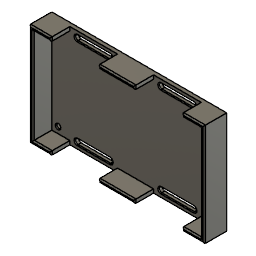
chassis_layer1_assembly_check_v0_1 (Autodesk Fusion 360 archive; units mm, degrees)
design "power_tray_v0_1_fusion_final"
part number: 2026-05-26-08-43-21-523
Autodesk Fusion 360 part; units mm, degrees
sketch "草图12" plane through (0, 0, 0) normal (0, 0, 1) x (1, 0, 0)
  line L0 (-69.75, -40.85) -> (69.75, -40.85)
  line L1 (69.75, -40.85) -> (69.75, 40.85)
  line L2 (69.75, 40.85) -> (-69.75, 40.85)
  line L3 (-69.75, 40.85) -> (-69.75, -40.85)
extrude "拉伸12" add sketch "草图12" along normal blind 3
ref_plane "工作平面2" through (0, 0, 3) normal (0, 0, 1) x (1, 0, 0)
sketch "草图13" plane through (0, 0, 3) normal (0, 0, 1) x (1, 0, 0)
  line L0 (-69.75, -40.85) -> (-66.75, -40.85)
  line L1 (-66.75, -40.85) -> (-66.75, 40.85)
  line L2 (-66.75, 40.85) -> (-69.75, 40.85)
  line L3 (-69.75, 40.85) -> (-69.75, -40.85)
extrude "拉伸13" add sketch "草图13" along normal blind 15
sketch "草图14" plane through (0, 0, 3) normal (0, 0, 1) x (1, 0, 0)
  line L0 (66.75, -40.85) -> (69.75, -40.85)
  line L1 (69.75, -40.85) -> (69.75, 40.85)
  line L2 (69.75, 40.85) -> (66.75, 40.85)
  line L3 (66.75, 40.85) -> (66.75, -40.85)
extrude "拉伸14" add sketch "草图14" along normal blind 15
sketch "草图15" plane through (0, 0, 3) normal (0, 0, 1) x (1, 0, 0)
  line L0 (-66.75, -40.85) -> (-52.375, -40.85)
  line L1 (-52.375, -40.85) -> (-52.375, -37.85)
  line L2 (-52.375, -37.85) -> (-66.75, -37.85)
  line L3 (-66.75, -37.85) -> (-66.75, -40.85)
extrude "拉伸15" add sketch "草图15" along normal blind 15
sketch "草图16" plane through (0, 0, 3) normal (0, 0, 1) x (1, 0, 0)
  line L0 (-14.375, -40.85) -> (14.375, -40.85)
  line L1 (14.375, -40.85) -> (14.375, -37.85)
  line L2 (14.375, -37.85) -> (-14.375, -37.85)
  line L3 (-14.375, -37.85) -> (-14.375, -40.85)
extrude "拉伸16" add sketch "草图16" along normal blind 15
sketch "草图17" plane through (0, 0, 3) normal (0, 0, 1) x (1, 0, 0)
  line L0 (52.375, -40.85) -> (66.75, -40.85)
  line L1 (66.75, -40.85) -> (66.75, -37.85)
  line L2 (66.75, -37.85) -> (52.375, -37.85)
  line L3 (52.375, -37.85) -> (52.375, -40.85)
extrude "拉伸17" add sketch "草图17" along normal blind 15
sketch "草图18" plane through (0, 0, 3) normal (0, 0, 1) x (1, 0, 0)
  line L0 (-66.75, 37.85) -> (-52.375, 37.85)
  line L1 (-52.375, 37.85) -> (-52.375, 40.85)
  line L2 (-52.375, 40.85) -> (-66.75, 40.85)
  line L3 (-66.75, 40.85) -> (-66.75, 37.85)
extrude "拉伸18" add sketch "草图18" along normal blind 15
sketch "草图19" plane through (0, 0, 3) normal (0, 0, 1) x (1, 0, 0)
  line L0 (-14.375, 37.85) -> (14.375, 37.85)
  line L1 (14.375, 37.85) -> (14.375, 40.85)
  line L2 (14.375, 40.85) -> (-14.375, 40.85)
  line L3 (-14.375, 40.85) -> (-14.375, 37.85)
extrude "拉伸19" add sketch "草图19" along normal blind 15
sketch "草图20" plane through (0, 0, 3) normal (0, 0, 1) x (1, 0, 0)
  line L0 (52.375, 37.85) -> (66.75, 37.85)
  line L1 (66.75, 37.85) -> (66.75, 40.85)
  line L2 (66.75, 40.85) -> (52.375, 40.85)
  line L3 (52.375, 40.85) -> (52.375, 37.85)
extrude "拉伸20" add sketch "草图20" along normal blind 15
sketch "草图21" plane through (0, 0, 3) normal (0, 0, 1) x (1, 0, 0)
  line L0 (-46.375, -33.85) -> (-20.375, -33.85)
  line L1 (-20.375, -37.85) -> (-46.375, -37.85)
  arc A0 (-20.375, -37.85) -> (-20.375, -33.85) centre (-20.375, -35.85) ccw
  arc A1 (-46.375, -33.85) -> (-46.375, -37.85) centre (-46.375, -35.85) ccw
  line L2 (-46.375, 37.85) -> (-20.375, 37.85)
  line L3 (-20.375, 33.85) -> (-46.375, 33.85)
  arc A2 (-20.375, 33.85) -> (-20.375, 37.85) centre (-20.375, 35.85) ccw
  arc A3 (-46.375, 37.85) -> (-46.375, 33.85) centre (-46.375, 35.85) ccw
  line L4 (20.375, -33.85) -> (46.375, -33.85)
  line L5 (46.375, -37.85) -> (20.375, -37.85)
  arc A4 (46.375, -37.85) -> (46.375, -33.85) centre (46.375, -35.85) ccw
  arc A5 (20.375, -33.85) -> (20.375, -37.85) centre (20.375, -35.85) ccw
  line L6 (20.375, 37.85) -> (46.375, 37.85)
  line L7 (46.375, 33.85) -> (20.375, 33.85)
  arc A6 (46.375, 33.85) -> (46.375, 37.85) centre (46.375, 35.85) ccw
  arc A7 (20.375, 37.85) -> (20.375, 33.85) centre (20.375, 35.85) ccw
extrude "拉伸21" cut sketch "草图21" against normal blind 3.2
sketch "草图22" plane through (0, 0, 3) normal (0, 0, 1) x (1, 0, 0)
  circle A0 centre (-61.75, -32.85) radius 1.6
  circle A1 centre (-61.75, 32.85) radius 1.6
  circle A2 centre (61.75, -32.85) radius 1.6
  circle A3 centre (61.75, 32.85) radius 1.6
extrude "拉伸22" cut sketch "草图22" against normal blind 3.2
fillet "圆角2" radius 1 24 edges at (59.5625, 37.85, 18) (52.375, 39.35, 18) (66.75, 0, 18) (14.375, 39.35, 18) (0, 37.85, 18) (-14.375, 39.35, 18) (0, 40.85, 18) (-52.375, 39.35, 18) (-59.5625, 37.85, 18) (59.5625, -37.85, 18) (52.375, -39.35, 18) (0, -37.85, 18) (14.375, -39.35, 18) (-14.375, -39.35, 18) (0, -40.85, 18) (-59.5625, -37.85, 18) (-52.375, -39.35, 18) (-66.75, 0, 18) (61.0625, -40.85, 18) (69.75, 0, 18) (61.0625, 40.85, 18) (-69.75, 0, 18) (-61.0625, -40.85, 18) (-61.0625, 40.85, 18)
fillet "圆角3" radius 0.6 68 edges at (60.2583, -32.2714, 3) (-63.2417, 33.4286, 3) (-63.2417, -32.2714, 3) (60.2583, 33.4286, 3) (33.375, -37.85, 3) (18.375, -35.85, 3) (33.375, -33.85, 3) (48.375, -35.85, 3) (48.375, -35.85, 3) (33.375, -37.85, 3) (18.375, -35.85, 3) (33.375, -33.85, 3) (33.375, -33.85, 3) (48.375, -35.85, 3) (33.375, -37.85, 3) (18.375, -35.85, 3) (18.375, -35.85, 3) (33.375, -33.85, 3) (48.375, -35.85, 3) (33.375, -37.85, 3) (-33.375, 33.85, 3) (-48.375, 35.85, 3) (-33.375, 37.85, 3) (-18.375, 35.85, 3) (-18.375, 35.85, 3) (-33.375, 33.85, 3) (-48.375, 35.85, 3) (-33.375, 37.85, 3) (-33.375, 37.85, 3) (-18.375, 35.85, 3) (-33.375, 33.85, 3) (-48.375, 35.85, 3) (-48.375, 35.85, 3) (-33.375, 37.85, 3) (-18.375, 35.85, 3) (-33.375, 33.85, 3) (-33.375, -37.85, 3) (-48.375, -35.85, 3) (-33.375, -33.85, 3) (-18.375, -35.85, 3) (-18.375, -35.85, 3) (-33.375, -37.85, 3) (-48.375, -35.85, 3) (-33.375, -33.85, 3) (-33.375, -33.85, 3) (-18.375, -35.85, 3) (-33.375, -37.85, 3) (-48.375, -35.85, 3) (-48.375, -35.85, 3) (-33.375, -33.85, 3) (-18.375, -35.85, 3) (-33.375, -37.85, 3) (33.375, 33.85, 3) (18.375, 35.85, 3) (33.375, 37.85, 3) (48.375, 35.85, 3) (48.375, 35.85, 3) (33.375, 33.85, 3) (18.375, 35.85, 3) (33.375, 37.85, 3) (33.375, 37.85, 3) (48.375, 35.85, 3) (33.375, 33.85, 3) (18.375, 35.85, 3) (18.375, 35.85, 3) (33.375, 37.85, 3) (48.375, 35.85, 3) (33.375, 33.85, 3)
sketch "草图7" plane through (0, 0, 3) normal (0, 0, 1) x (1, 0, 0)
  line L0 (-66.75, 37.85) -> (-52.375, 37.85)
  line L1 (-52.375, 37.85) -> (-52.375, 40.85)
  line L2 (-52.375, 40.85) -> (-66.75, 40.85)
  line L3 (-66.75, 40.85) -> (-66.75, 37.85)
sketch "草图8" plane through (0, 0, 3) normal (0, 0, 1) x (1, 0, 0)
  line L0 (-14.375, 37.85) -> (14.375, 37.85)
  line L1 (14.375, 37.85) -> (14.375, 40.85)
  line L2 (14.375, 40.85) -> (-14.375, 40.85)
  line L3 (-14.375, 40.85) -> (-14.375, 37.85)
sketch "草图9" plane through (0, 0, 3) normal (0, 0, 1) x (1, 0, 0)
  line L0 (52.375, 37.85) -> (66.75, 37.85)
  line L1 (66.75, 37.85) -> (66.75, 40.85)
  line L2 (66.75, 40.85) -> (52.375, 40.85)
  line L3 (52.375, 40.85) -> (52.375, 37.85)
sketch "草图10" plane through (0, 0, 3) normal (0, 0, 1) x (1, 0, 0)
  line L0 (-46.375, -33.85) -> (-20.375, -33.85)
  line L1 (-20.375, -37.85) -> (-46.375, -37.85)
  arc A0 (-20.375, -37.85) -> (-20.375, -33.85) centre (-20.375, -35.85) ccw
  arc A1 (-46.375, -33.85) -> (-46.375, -37.85) centre (-46.375, -35.85) ccw
  line L2 (-46.375, 37.85) -> (-20.375, 37.85)
  line L3 (-20.375, 33.85) -> (-46.375, 33.85)
  arc A2 (-20.375, 33.85) -> (-20.375, 37.85) centre (-20.375, 35.85) ccw
  arc A3 (-46.375, 37.85) -> (-46.375, 33.85) centre (-46.375, 35.85) ccw
  line L4 (20.375, -33.85) -> (46.375, -33.85)
  line L5 (46.375, -37.85) -> (20.375, -37.85)
  arc A4 (46.375, -37.85) -> (46.375, -33.85) centre (46.375, -35.85) ccw
  arc A5 (20.375, -33.85) -> (20.375, -37.85) centre (20.375, -35.85) ccw
  line L6 (20.375, 37.85) -> (46.375, 37.85)
  line L7 (46.375, 33.85) -> (20.375, 33.85)
  arc A6 (46.375, 33.85) -> (46.375, 37.85) centre (46.375, 35.85) ccw
  arc A7 (20.375, 37.85) -> (20.375, 33.85) centre (20.375, 35.85) ccw
sketch "草图11" plane through (0, 0, 3) normal (0, 0, 1) x (1, 0, 0)
  circle A0 centre (-61.75, -32.85) radius 1.6
  circle A1 centre (-61.75, 32.85) radius 1.6
  circle A2 centre (61.75, -32.85) radius 1.6
  circle A3 centre (61.75, 32.85) radius 1.6
named bodies: "power_tray_body"

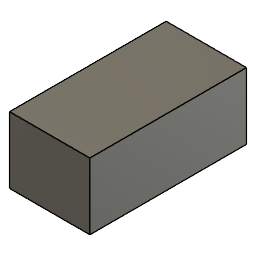
design "电池"
part number: 2026-05-28-00-42-13-153
Autodesk Fusion 360 part; units mm, degrees
box "长方体基本要素1" add length 132 width 67.7 height 56 placed x (0, 0, 1) y (1, 0, 0) z (0, 1, 0) at (0, 0, 0)

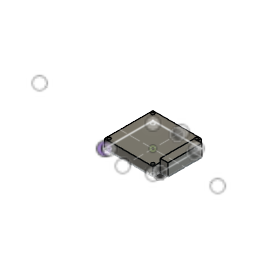
design "电驱"
part number: 2026-05-28-00-46-10-485
Autodesk Fusion 360 part; units mm, degrees
sketch "草图1" plane through (0, 0, 0) normal (0, 1, 0) x (1, 0, 0)
  line L0 (0, 0) -> (50, 0)
  line L1 (50, 0) -> (50, 50)
  line L2 (50, 50) -> (0, 50)
  line L3 (0, 50) -> (0, 0)
  line L4 (0, 0) -> (50, 0)
  line L5 (58, 7.5) -> (58, 42.5)
  line L6 (50, 50) -> (0, 50)
  line L7 (0, 50) -> (0, 0)
  circle A0 centre (47.5, 47.5) radius 1.6
  line L8 (-91.8242, 25) -> (91.8242, 25) construction
  circle A1 centre (2.5, 47.5) radius 1.6
  circle A2 centre (2.5, 2.5) radius 1.6
  circle A3 centre (47.5, 2.5) radius 1.6
  line L9 (25, 54.7536) -> (25, -6.1095) construction
  line L10 (50, 42.5) -> (58, 42.5)
  line L11 (50, 7.5) -> (58, 7.5)
  point P0 (25, 50)
  point P1 (25, 25)
  point P2 (50, 42.5)
  point P3 (50, 7.5)
  dimension "d1" = 50
  dimension "d2" = 50
  dimension "d4" = 50
  dimension "d5" = 3.2
  dimension "d6" = 45
  dimension "d7" = 45
  dimension "d8" = 35
  dimension "d9" = 8
  constraint horizontal L0
  constraint vertical L1
  constraint horizontal L2
  constraint vertical L3
  constraint coincident L0.start L3.end
  constraint horizontal L4
  constraint vertical L5
  constraint horizontal L6
  constraint vertical L7
  constraint horizontal L8
  constraint midpoint L3 L8
  constraint equal A0 A1
  constraint equal A0 A2
  constraint equal A0 A3
  constraint coincident L6 P0
  constraint midpoint L2 P0
  constraint perpendicular L0 L9
  constraint coincident L8 P1
  constraint coincident L9 P1
  constraint symmetric A0.centre A1.centre L9
  constraint symmetric A2.centre A3.centre L9
  constraint symmetric L8 A1.centre A2.centre
  constraint coincident L1 P2
  constraint coincident L1 P3
  constraint symmetric L8 P2 P3
  constraint coincident P2 L10.start
  constraint perpendicular L5 L10
  constraint coincident P3 L11.start
  constraint perpendicular L5 L11
  measures "d1" distance of L0.start L0.end
  measures "d2" distance of L0.start L2.end
  measures "d4" distance of L0.start L2.end
  measures "d5" diameter of A0
  measures "d6" distance of A0.centre A1.centre
  measures "d7" distance of A1.centre A2.centre
  measures "d8" distance of P2 P3
  measures "d9" distance of P3 L5.start
extrude "拉伸1" add sketch "草图1" along normal blind 9 contours L0 L1 L2 L3 L4 L6 L7
extrude "拉伸2" add sketch "草图1" along normal blind 12.6 contours L1 L5 L10 L11

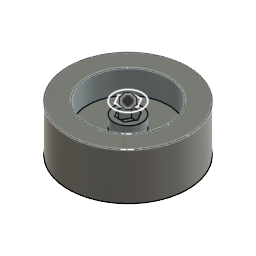
design "轮胎"
part number: 2026-05-27-21-11-46-557
Autodesk Fusion 360 part; units mm, degrees
sketch "草图1" plane through (0, 0, 0) normal (0, 1, 0) x (1, 0, 0)
  circle A0 centre (0, 0) radius 42.5
  circle A1 centre (0, 0) radius 28.8
  circle A2 centre (0, 0) radius 10
  line L0 (-3.4641, 6) -> (3.4641, 6)
  line L1 (3.4641, 6) -> (6.9282, 0)
  line L2 (6.9282, 0) -> (3.4641, -6)
  line L3 (3.4641, -6) -> (-3.4641, -6)
  line L4 (-3.4641, -6) -> (-6.9282, 0)
  line L5 (-6.9282, 0) -> (-3.4641, 6)
  line L6 (0, 6) -> (0, -6) construction
  dimension "d1" = 85
  dimension "d2" = 57.6
  dimension "d3" = 20
  dimension "d11" = 120
  dimension "d12" = 120
  dimension "d13" = 12
  constraint coincident A0.centre A1.centre
  constraint concentric A0 A1
  constraint concentric A1 A2
  constraint horizontal L0
  constraint parallel L0 L3
  constraint equal L0 L1
  constraint equal L0 L2
  constraint equal L0 L3
  constraint equal L0 L4
  constraint equal L0 L5
  constraint coincident L0 L6.start
  constraint coincident L3 L6.end
  constraint perpendicular L3 L6
  constraint midpoint L6 A0.centre
  constraint symmetric L1 L5 L6
  measures "d1" diameter of A0
  measures "d2" diameter of A1
  measures "d3" diameter of A2
  measures "d11" angle of L4 L5
  measures "d12" angle of L0 L1
  measures "d13" distance of L0 L3
extrude "拉伸1" add sketch "草图1" against normal blind 33.4 contours A0 | A1 | A2 | L0 L1 L2 L3 L4 L5
extrude "拉伸2" cut sketch "草图1" against normal blind 17 contours A1
extrude "拉伸3" cut sketch "草图1" against normal blind 8.3 contours A2 | L0 L1 L2 L3 L4 L5
extrude "拉伸4" cut sketch "草图1" against normal blind 15.3 contours L0 L1 L2 L3 L4 L5
equation "d14 = -7 mm - 8.3 mm"

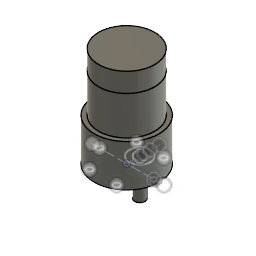
design "电机"
part number: 2026-05-27-19-27-58-394
Autodesk Fusion 360 part; units mm, degrees
cylinder "圆柱体基本要素1" add diameter 37 height 24 placed x (1, 0, 0) y (0, 0, -1) z (0, 1, 0) at (0, 0, 0) makes body 1
cylinder "圆柱体基本要素2" add diameter 32 height 22 placed x (1, 0, 0) y (0, 0, -1) z (0, 1, 0) at (0, 24, 0) bodies 1
cylinder "圆柱体基本要素3" add diameter 32 height 11 placed x (1, 0, 0) y (0, 0, -1) z (0, 1, 0) at (0, 46, 0) separate body makes body 2
sketch "草图5" plane through (0, 0, 0) normal (0, -1, 0) x (1, 0, 0)
  circle A0 centre (0, 0) radius 18.5
  line L0 (0, 0) -> (0, -18.5) construction
  circle A1 centre (0, -7.5) radius 6
  line L1 (1.6583, -10) -> (-1.6583, -10)
  arc A2 (1.6583, -10) -> (-1.6583, -10) centre (0, -7.5) ccw
  circle A3 centre (0, -7.5) radius 3
  circle A4 centre (-15.5, 0) radius 1.6
  circle A5 centre (-7.75, -13.4234) radius 1.6
  circle A6 centre (7.75, -13.4234) radius 1.6
  circle A7 centre (15.5, 0) radius 1.6
  circle A8 centre (7.75, 13.4234) radius 1.6
  circle A9 centre (-7.75, 13.4234) radius 1.6
  line L2 (-19.7514, 0) -> (21.2486, 0) construction
  point P0 (0, -18.5)
  point P1 (0, -7.5)
  point P2 (0, -10)
  point P3 (0, -13.5)
  dimension "d10" = 12
  dimension "d11" = 6
  dimension "d12" = 2.5
  dimension "d13" = 5
  dimension "d20" = 3.2
  dimension "d22" = 360
  dimension "d23" = 31
  constraint coincident A0 P0
  constraint coincident A0.centre L0.start
  constraint coincident P0 L0.end
  constraint coincident L0 P1
  constraint coincident P1 A1.centre
  constraint coincident L0 P2
  constraint perpendicular L0 L1
  constraint coincident P2 L1
  constraint coincident A1 P3
  constraint coincident L0 P3
  constraint concentric A1 A3
  constraint vertical L0
  constraint horizontal L2
  constraint coincident A0.centre L2
  constraint coincident A7.centre L2
  measures "d10" diameter of A1
  measures "d11" diameter of A2
  measures "d12" distance of P1 P2
  measures "d13" distance of P0 P3
  measures "d20" diameter of A4
  measures "d23" distance of A4.centre A7.centre
extrude "拉伸1" add sketch "草图5" along normal blind 6 contours A1 | L1 A3 bodies 1
extrude "拉伸2" add 1 faces at (-0.2173, 0, -8.1906) along direction (0, -1, 0) blind 21 on bodies 1 bodies 1
sketch "草图6" plane through (0, -6, 0) normal (0, -1, 0) x (1, 0, 0)
  arc A0 (1.6583, -10) -> (-1.6583, -10) centre (0, -7.5) ccw
  line L0 (1.6583, -10) -> (-1.6583, -10)
  circle A1 centre (0, -7.5) radius 6
extrude "拉伸3" add sketch "草图5" along normal blind 9 contours L1 A3 | L1 A2 A3 bodies 1

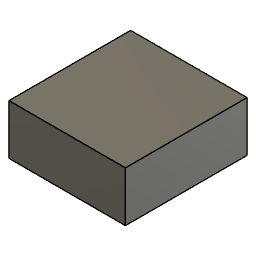
design "保险盒"
part number: 2026-05-28-09-32-34-860
Autodesk Fusion 360 part; units mm, degrees
box "长方体基本要素1" add length 88 width 84.2 height 36.2 placed x (0, 0, 1) y (1, 0, 0) z (0, 1, 0) at (0, 0, 0)
sketch "草图2" plane through (0, 0, 0) normal (0, -1, 0) x (1, 0, 0)
  line L0 (84.2, 88) -> (0, 88)
  line L1 (0, 88) -> (0, 0)
  line L2 (0, 0) -> (84.2, 0)
  line L3 (84.2, 0) -> (84.2, 88)
  line L4 (42.1, 88) -> (42.1, -8.9245) construction
  line L5 (0, 44) -> (89.0671, 44) construction
  circle A0 centre (7.2, 80.85) radius 2
  circle A1 centre (7.2, 7.15) radius 2
  circle A2 centre (77, 7.15) radius 2
  circle A3 centre (77, 80.85) radius 2
  point P0 (42.1, 88)
  point P1 (0, 44)
  dimension "d8" = 4
  dimension "d9" = 73.7
  dimension "d10" = 69.8
  constraint midpoint L0 P0
  constraint midpoint L1 P1
  constraint coincident P0 L4.start
  constraint perpendicular L0 L4
  constraint coincident P1 L5.start
  constraint perpendicular L3 L5
  constraint equal A0 A3
  constraint equal A0 A2
  constraint equal A0 A1
  constraint symmetric L5 A0.centre A1.centre
  constraint symmetric L4 A0.centre A3.centre
  constraint symmetric L5 A2.centre A3.centre
  measures "d8" diameter of A0
  measures "d9" distance of A0.centre A1.centre
  measures "d10" distance of A0.centre A3.centre
extrude "拉伸1" cut sketch "草图2" against normal blind 12.3 contours A0 | A1 | A2 | A3

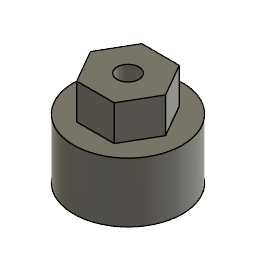
design "联轴器"
part number: 2026-05-27-20-20-33-516
Autodesk Fusion 360 part; units mm, degrees
cylinder "圆柱体基本要素1" add diameter 20 height 11 placed x (1, 0, 0) y (0, 0, -1) z (0, 1, 0) at (0, 0, 0)
sketch "草图2" plane through (0, 11, 0) normal (0, 1, 0) x (-1, 0, 0)
  circle A0 centre (0, 0) radius 10
  line L0 (3.4641, -6) -> (-3.4641, -6)
  line L1 (-3.4641, -6) -> (-6.9282, 0)
  line L2 (-6.9282, 0) -> (-3.4641, 6)
  line L3 (-3.4641, 6) -> (3.4641, 6)
  line L4 (3.4641, 6) -> (6.9282, 0)
  line L5 (6.9282, 0) -> (3.4641, -6)
  line L6 (3.4641, -6) -> (-3.4641, 6) construction
  dimension "d4" = 12
  dimension "d5" = 120
  dimension "d6" = 120
  constraint horizontal L0
  constraint parallel L0 L3
  constraint parallel L1 L4
  constraint parallel L2 L5
  constraint equal L0 L1
  constraint equal L1 L2
  constraint equal L1 L3
  constraint equal L1 L4
  constraint midpoint L6 A0.centre
  constraint coincident A0.centre origin
  measures "d4" distance of L0 L3
  measures "d5" angle of L0 L5
  measures "d6" angle of L1 L2
extrude "拉伸1" add sketch "草图2" along normal blind 6.5 contours L0 L1 L2 L3 L4 L5
cylinder "圆柱体基本要素2" cut diameter 4 height -5.7 placed x (1, 0, 0) y (0, 0, -1) z (0, 1, 0) at (0, 17.5, 0)
cylinder "圆柱体基本要素3" cut diameter 6 height -11.8 placed x (1, 0, 0) y (0, 0, -1) z (0, 1, 0) at (0, 11.8, 0)
